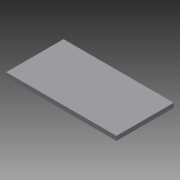
# Autodesk Inventor part: pala
Saved by Autodesk Inventor 2015 (Build 190159000, 159)
## iProperties
Created: 2015-02-22
Part Number: pala
Material: Genérico
Document SubType Name: Modeling
Designer: jorge
Density: 1 g/cm^3
Appearance: Valor por defecto
Author: jorge
Autodesk Inventor part; units mm, degrees
ref_plane "YZ Plane" through (0, 0, 0) normal (1, 0, 0) x (0, 1, 0)
ref_plane "XZ Plane" through (0, 0, 0) normal (0, 1, 0) x (-1, 0, 0)
ref_plane "XY Plane" through (0, 0, 0) normal (0, 0, 1) x (1, 0, 0)
sketch "Boceto1" plane through (0, 0, 0) normal (0, 0, 1) x (1, 0, 0)
  line L0 (0, 0) -> (-127, 0) projected
  line L1 (-3, -66) -> (-124, -66) projected
  line L2 (-127, 0) -> (0, 0)
  line L3 (0, 0) -> (0, -66)
  line L4 (0, -66) -> (-127, -66)
  line L5 (-127, -66) -> (-127, 0)
  constraints: 8 end point, 2 parallel, 1 horizontal, 1 perpendicular
extrude "Extrusión1" add sketch "Boceto1" along normal blind 5
move faces "Desplazar1" translate (-7.7586, 0, 0) faces at (-127, -44, 1.6667)
sketch "Boceto3" plane through (-134.7586, -66, 0) normal (-1, 0, 0) x (0, 0, 1)
  line L0 (-19.6414, 77.5) -> (-19.6414, 74.1) projected
  line L1 (-22.2414, 74.1) -> (-22.2414, 77.5) projected
  line L2 (-22.2414, 66.1) -> (-22.2414, 69.5) projected
  line L3 (-19.6414, 69.5) -> (-19.6414, 66.1) projected
  line L4 (-15.2414, 70.5) -> (-18.6414, 70.5) projected
  line L5 (-18.6414, 73.1) -> (-15.2414, 73.1) projected
  line L6 (-26.6414, 73.1) -> (-23.2414, 73.1) projected
  line L7 (-23.2414, 70.5) -> (-26.6414, 70.5) projected
  arc A0 (-19.6414, 77.5) -> (-22.2414, 77.5) centre (-20.9414, 77.5) ccw projected
  arc A1 (-22.2414, 66.1) -> (-19.6414, 66.1) centre (-20.9414, 66.1) ccw projected
  line L8 (5, 66) -> (5, 78.8)
  line L9 (5, 66) -> (5, 64.8)
  line L10 (5, 78.8) -> (5, 49.624)
  line L11 (5, 66) -> (5, 0) projected
  arc A2 (-19.6414, 79.5) -> (-22.2414, 79.5) centre (-20.9414, 79.5) ccw projected
  arc A3 (-22.2414, 68.1) -> (-19.6414, 68.1) centre (-20.9414, 68.1) ccw projected
  line L12 (5, 49.624) -> (5, 51.624)
  line L13 (5, 51.624) -> (-20.9414, 66.8)
  line L14 (5, 78.8) -> (5, 80.8)
  line L15 (5, 80.8) -> (-20.9414, 80.8)
  circle A4 centre (-20.9414, 73.8) radius 0.75 projected
  arc A5 (-20.9414, 80.8) -> (-20.9414, 66.8) centre (-20.9414, 73.8) ccw
  circle A6 centre (-20.9414, 73.8) radius 1.45 projected
  circle A7 centre (-20.9414, 78.95) radius 0.5 projected
  point P0 (0, 66)
  point P1 (-20.9414, 71.8)
  point P2 (-20.9414, 78.8)
  dimension "d28" = 29.176
  dimension "d29" = 2
  dimension "d30" = 2
  constraints: 14 end point, 5 point on circle, 3 point on line, 3 vertical, 1 centre point, 1 coincident, 1 other
  measures "d28" distance of L8.end L10.end
  measures "d29" distance of L10.end L12.end
  measures "d30" distance of L8.end L14.end
extrude "Extrusión2" add sketch "Boceto3" along normal blind 4 contours L0 A6 L1 A0 A7 | A6 | A7 A0 | A0 A7 | A5 L15 L14 L8 L9 L10 L13 A1 L3 A3 L2 | L2 A3 A5 | L13 A3 L3 A1 | A4
move faces "Desplazar2" translate (-4, 0, 0) faces at (-134.7586, -30.609, 1.6667)
sketch "Boceto4" plane through (-138.7586, -66, 0) normal (-1, 0, 0) x (0, 0, 1)
  circle A0 centre (-15.7914, 73.8) radius 0.5 projected
  circle A1 centre (-20.9414, 68.65) radius 0.5 projected
  circle A2 centre (-26.0914, 73.8) radius 0.5 projected
  circle A3 centre (-20.9414, 78.95) radius 0.5 projected
  circle A4 centre (-20.9414, 78.95) radius 0.5 projected
  circle A5 centre (-20.9414, 78.95) radius 0.5 projected
  point P0 (0, 66)
hole "Agujero1" at (-138.7586, 7.8, -15.7914) at (-138.7586, 2.65, -20.9414) at (-138.7586, 7.8, -26.0914) direction (1, 0, 0) diameter 2 end up to face face through (-134.7586, 9.8667, -5.3138) facing (1, 0, 0)
ref_plane "Plano de trabajo1" through (0, 0, -79) normal (1, 0, 0) x (0, 0, -1)
offset faces "Tamaño1" outward 5 faces at (0, -22, 1.6667)
sketch "Boceto6" plane through (5, -66, 0) normal (1, 0, 0) x (0, 0, -1)
  arc A0 (20.9414, 64.8) -> (20.9414, 78.8) centre (20.9414, 71.8) ccw projected
  line L0 (-5, 78.8) -> (20.9414, 78.8) projected
  line L1 (-5, 78.8) -> (-5, 66) projected
  line L2 (-5, 0) -> (-5, 66) projected
  line L3 (0, 49.6235) -> (20.9414, 64.8) projected
  line L4 (0, 49.6235) -> (-5, 49.6235)
  line L5 (-5, 0) -> (-5, 66) projected
  point P0 (0, 66)
  constraints: 2 end point, 1 perpendicular, 1 point on line
extrude "Extrusión3" add sketch "Boceto6" against normal blind 4
sketch "Boceto7" plane through (5, -66, 5) normal (1, 0, 0) x (0, 0, -1)
  circle A0 centre (25.9414, 73.8) radius 1.45 projected
  point P0 (5, 66)
hole "Agujero2" at (5, 7.8, -20.9414) direction (-1, 0, 0) diameter 9 end up to face face through (1, -5.8588, -6.9805) facing (-1, 0, 0)
hole "Agujero3" at (-138.7586, 7.8, -20.9414) direction (1, 0, 0) diameter 2 depth 2 tip angle 118
sketch "Boceto9" plane through (-138.7586, -66, 0) normal (-1, 0, 0) x (0, 0, 1)
  circle A0 centre (-20.9414, 78.95) radius 0.5 projected
  point P0 (0, 66)
hole "Agujero4" at (-138.7586, 12.95, -20.9414) direction (1, 0, 0) diameter 2 end up to face face through (-134.7586, 7.6131, -3.2735) facing (1, 0, 0)
sketch "Boceto10" plane through (5, -66, 5) normal (1, 0, 0) x (0, 0, -1)
  circle A0 centre (49.5, 31.4977) radius 40 projected
  line L0 (49.5, -8.5023) -> (-0.0805, -8.5023)
  line L1 (-0.0805, -8.5023) -> (5, -8.5023)
  line L2 (5, -8.5023) -> (5, 0)
  line L3 (5, 0) -> (-0.0805, 0)
  line L4 (-0.0805, 0) -> (-0.0805, -8.5023)
  point P0 (5, 66)
  constraints: 10 end point, 2 horizontal, 2 parallel, 1 perpendicular, 1 vertical alignment, 1 other
extrude "Extrusión4" add sketch "Boceto10" against normal up to surface (143.7586 mm away) contours L0 L4 L3 L2
